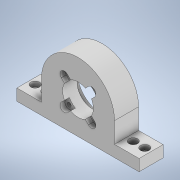
# Autodesk Inventor part: Motor_bracket
Saved by Autodesk Inventor 2020 (Build 240168000, 168)
## iProperties
Created: 2022-06-09
Part Number: Motor_bracket
Material: 일반
Document SubType Name: Modeling
Designer: samsung
Density: 1 g/cm^3
Appearance: 기본값
Author: samsung
Autodesk Inventor part; units mm, degrees
ref_plane "YZ Plane" through (0, 0, 0) normal (1, 0, 0) x (0, 1, 0)
ref_plane "XZ Plane" through (0, 0, 0) normal (0, 1, 0) x (-1, 0, 0)
ref_plane "작업 평면1" through (0, 0, 0) normal (0, 0, 1) x (1, 0, 0)
sketch "스케치1" plane through (0, 0, 0) normal (0, 0, 1) x (1, 0, 0)
  circle A0 centre (0, 0) radius 26 projected
  circle A1 centre (0, 0) radius 16 projected
  line L0 (25, -33.3) -> (-25, -33.3) projected
  line L1 (-63.5, -33.3) -> (63.5, -33.3)
  line L2 (63.5, -33.3) -> (63.5, -21.3)
  line L3 (-63.5, -21.3) -> (-63.5, -33.3)
  arc A2 (38, 0) -> (-38, 0) centre (0, 0) ccw
  line L4 (-38, 0) -> (-38, -21.3)
  line L5 (38, 0) -> (38, -21.3)
  line L6 (63.5, -21.3) -> (38, -21.3)
  line L7 (-38, -21.3) -> (-63.5, -21.3)
  point P0 (0, -33.3)
  dimension "d1" = 12
  dimension "d11" = 12
  dimension "d14" = 127
  dimension "d67" = 76
  dimension "d68" = 25.5
  dimension "d69" = 25.5
  dimension "d70" = 21.3
  dimension "d79" = 32
  dimension "d80" = 52
  constraints: 14 end point, 3 horizontal, 2 midpoint, 2 point on circle, 2 vertical, 1 centre point, 1 parallel, 1 perpendicular, 1 tangent
  measures "d1" distance of L2.end L1.end
  measures "d11" distance of L3.start L1.start
  measures "d14" distance between parallel lines of L2 L3
  measures "d67" diameter of A2
  measures "d68" distance of L2.end L5.end
  measures "d69" distance of L4.end L3.start
  measures "d70" distance of L4.start L4.end
  measures "d79" diameter of A1
  measures "d80" diameter of A0
extrude "돌출1" add sketch "스케치1" along normal blind 15 contours A0 | L0 L1 L3 L7 L4 A2 L5 L6 L2
sketch "스케치5" plane through (0, 0, 0) normal (0, 0, -1) x (-1, 0, 0)
  circle A0 centre (0, 0) radius 26 projected
  line L0 (63.5, -33.3) -> (-63.5, -33.3) projected
  line L1 (63.5, -21.3) -> (63.5, -33.3) projected
  line L2 (-63.5, -33.3) -> (-63.5, -21.3) projected
  line L3 (-63.5, -21.3) -> (-63.5, -33.3)
  line L4 (-63.5, -33.3) -> (63.5, -33.3)
  line L5 (63.5, -33.3) -> (63.5, -21.3)
  circle A1 centre (0, 0) radius 26
  arc A2 (38, 0) -> (-38, 0) centre (0, 0) ccw projected
  line L6 (-38, -21.3) -> (-38, 0) projected
  line L7 (-63.5, -21.3) -> (-38, -21.3) projected
  line L8 (-63.5, -33.3) -> (-63.5, -21.3) projected
  line L9 (63.5, -33.3) -> (-63.5, -33.3) projected
  line L10 (63.5, -21.3) -> (63.5, -33.3) projected
  line L11 (38, -21.3) -> (63.5, -21.3) projected
  line L12 (38, 0) -> (38, -21.3) projected
  circle A3 centre (0, 0) radius 16 projected
  arc A4 (38, 0) -> (-38, 0) centre (0, 0) ccw
  line L13 (-38, -21.3) -> (-38, 0) projected
  line L14 (-38, 0) -> (-38, -21.3)
  line L15 (-38, -21.3) -> (-63.5, -21.3)
  line L16 (38, 0) -> (38, -21.3)
  constraints: 12 end point, 3 perpendicular, 2 centre point, 2 coincident, 2 point on circle, 2 vertical, 1 collinear, 1 concentric, 1 point on line
extrude "돌출3" add sketch "스케치5" along normal blind 10 contours L0 L2 L7 L6 A2 L12 L11 L1
sketch "스케치9" plane through (0, 0, 15) normal (0, 0, 1) x (1, 0, 0)
  circle A0 centre (0, 0) radius 20
  point P0 (-14.1421, 14.1421)
  point P1 (14.1421, 14.1421)
  point P2 (14.1421, -14.1421)
  point P3 (-14.1421, -14.1421)
  constraints: 1 coincident, 3 other
hole "구멍3" at (-14.1421, 14.1421, 15) at (14.1421, 14.1421, 15) at (14.1421, -14.1421, 15) at (-14.1421, -14.1421, 15) direction (0, 0, -1) diameter 4.134 end through all counterbore diameter 9 counterbore depth 5 thread size "M5x0.8" class "6H" standard "ISO Metric profile"
sketch "스케치11" plane through (0, 0, 15) normal (0, 0, 1) x (1, 0, 0)
  arc A0 (-9.9369, 12.5403) -> (-12.5403, 9.9369) centre (-14.1421, 14.1421) ccw projected
  arc A1 (12.5403, 9.9369) -> (9.9369, 12.5403) centre (14.1421, 14.1421) ccw projected
  arc A2 (9.9369, -12.5403) -> (12.5403, -9.9369) centre (14.1421, -14.1421) ccw projected
  arc A3 (-12.5403, -9.9369) -> (-9.9369, -12.5403) centre (-14.1421, -14.1421) ccw projected
  arc A4 (9.9369, 12.5403) -> (-9.9369, 12.5403) centre (0, 0) ccw projected
  arc A5 (12.5403, -9.9369) -> (12.5403, 9.9369) centre (0, 0) ccw projected
  arc A6 (-12.5403, 9.9369) -> (-12.5403, -9.9369) centre (0, 0) ccw projected
  arc A7 (-9.9369, -12.5403) -> (9.9369, -12.5403) centre (0, 0) ccw projected
  circle A8 centre (0, 0) radius 16
  line L0 (14.1421, 14.1421) -> (10.9602, 17.3241)
  line L1 (14.1421, 14.1421) -> (17.3241, 10.9602)
  line L2 (14.3241, 20.6881) -> (20.6881, 14.3241)
  line L3 (20.6881, 14.3241) -> (13.9602, 7.5962)
  line L4 (13.9602, 7.5962) -> (7.5962, 13.9602)
  line L5 (7.5962, 13.9602) -> (14.3241, 20.6881)
  line L6 (14.3241, 20.6881) -> (13.9602, 7.5962) construction
  line L7 (20.6881, 14.3241) -> (7.5962, 13.9602) construction
  line L8 (-14.1421, 14.1421) -> (-10.9602, 17.3241)
  line L9 (-14.1421, 14.1421) -> (-17.3241, 10.9602)
  line L10 (-20.6535, 14.2896) -> (-14.2896, 20.6535)
  line L11 (-14.2896, 20.6535) -> (-7.6307, 13.9947)
  line L12 (-7.6307, 13.9947) -> (-13.9947, 7.6307)
  line L13 (-13.9947, 7.6307) -> (-20.6535, 14.2896)
  line L14 (-20.6535, 14.2896) -> (-7.6307, 13.9947) construction
  line L15 (-14.2896, 20.6535) -> (-13.9947, 7.6307) construction
  line L16 (-14.1421, -14.1421) -> (-17.3241, -10.9602)
  line L17 (-14.1421, -14.1421) -> (-10.9602, -17.3241)
  line L18 (14.1421, -14.1421) -> (17.3241, -10.9602)
  arc A9 (9.9369, -12.5403) -> (12.5403, -9.9369) centre (14.1421, -14.1421) ccw projected
  line L19 (14.1421, -14.1421) -> (10.9602, -17.3241)
  line L20 (-20.6535, -14.2896) -> (-14.2896, -20.6535)
  line L21 (-14.2896, -20.6535) -> (-7.6307, -13.9947)
  line L22 (-7.6307, -13.9947) -> (-13.9947, -7.6307)
  line L23 (-13.9947, -7.6307) -> (-20.6535, -14.2896)
  line L24 (-20.6535, -14.2896) -> (-7.6307, -13.9947) construction
  line L25 (-14.2896, -20.6535) -> (-13.9947, -7.6307) construction
  line L26 (14.2554, -20.6193) -> (20.6193, -14.2554)
  line L27 (20.6193, -14.2554) -> (14.0289, -7.665)
  line L28 (14.0289, -7.665) -> (7.665, -14.0289)
  line L29 (7.665, -14.0289) -> (14.2554, -20.6193)
  line L30 (14.2554, -20.6193) -> (14.0289, -7.665) construction
  line L31 (20.6193, -14.2554) -> (7.665, -14.0289) construction
  point P0 (0, 0)
  point P1 (7.675, -14.039)
  point P2 (14.039, -7.675)
  point P3 (-7.675, -14.039)
  point P4 (-14.039, -7.675)
  point P5 (14.039, 7.675)
  point P6 (7.675, 14.039)
  point P7 (-14.039, 7.675)
  point P8 (-7.675, 14.039)
  constraints: 64 end point, 10 parallel, 8 midpoint, 8 point on circle, 5 perpendicular, 4 point on line, 1 centre point, 1 coincident
extrude "돌출4" cut sketch "스케치11" against normal blind 5 contours A0 L11 A4 | A6 L13 A0 | L5 A1 A4 | A6 A3 L23 | A1 L3 A5 | A7 L21 A3 | L27 A2 A5 | A7 A2 L29
sketch "스케치12" plane through (-63.5, -21.3, 15) normal (0, 1, 0) x (1, 0, 0)
  line L0 (0, 0) -> (25, 0)
  line L1 (25, 0) -> (25, 25)
  line L2 (25, 25) -> (0, 25)
  line L3 (0, 25) -> (0, 0)
  line L4 (127, 0) -> (102, 0)
  line L5 (102, 0) -> (102, 25)
  line L6 (102, 25) -> (127, 25)
  line L7 (127, 25) -> (127, 0)
  point P0 (63.5, 15)
  point P1 (18.5, 12.5)
  point P2 (108.5, 12.5)
  point P3 (120.5, 12.5)
  point P4 (6.5, 12.5)
  dimension "d71" = 25
  dimension "d72" = 25
  dimension "d73" = 6.5
  dimension "d74" = 6.5
  dimension "d75" = 25
  dimension "d76" = 25
  dimension "d77" = 6.5
  dimension "d78" = 6.5
  constraints: 16 end point, 4 parallel, 2 horizontal, 2 perpendicular
  measures "d71" distance of L2.end L1.end
  measures "d72" distance of L2.end L0.start
  measures "d73" distance from line of L3 point (6.5, 12.5)
  measures "d74" distance from line of point (18.5, 12.5) L1
  measures "d75" distance of L5.end L6.end
  measures "d76" distance of L6.end L4.start
  measures "d77" distance from line of point (120.5, 12.5) L7
  measures "d78" distance from line of point (108.5, 12.5) L5
hole "구멍5" at (-45, -21.3, 2.5) at (45, -21.3, 2.5) at (57, -21.3, 2.5) at (-57, -21.3, 2.5) direction (0, -1, 0) diameter 4.134 end through all counterbore diameter 9 counterbore depth 5 thread size "M5x0.8" class "6H" standard "ISO Metric profile"
